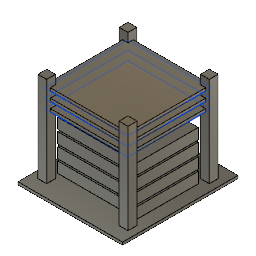
Mechanical Team Design 3Boards v2 (Autodesk Fusion 360 design; units mm, degrees)
Autodesk Fusion 360 part; units mm, degrees
box "BoxPrimitive1" add length 50 width 50 height 50 placed x (0, 0, 1) y (1, 0, 0) z (0, 1, 0) at (-20, 0, 10) makes body 1
box "BoxPrimitive2" add length 1.6 width 58 height 64 placed x (0, 0, -1) y (-1, 0, 0) z (0, 1, 0) at (33, 0, -10) separate body makes body 2
move_face "MoveFace1" by (10, 0, 0) 2 faces at (13.6667, 21.3333, -10) (-5.6667, 0, -10.5333) on bodies 2
move_body "Move1" bodies 2 to x (1, 0, 0) y (0, 1, 0) z (0, 0, 1) at (0, 0, 20)
move_face "MoveFace2" by (0, 5, 0) 1 faces at (13.6667, 21.3333, 10) on bodies 2
move_body "Move2" bodies 2 to x (1, 0, 0) y (0, 1, 0) z (0, 0, 1) at (0, -7, 0)
move_body "Move3" bodies 2 to x (1, 0, 0) y (0, 1, 0) z (0, 0, 1) at (5, 0, 0)
move_body "Move4" bodies 2 to x (1, 0, 0) y (0, 1, 0) z (0, 0, 1) at (-4, 0, 0)
sketch "Sketch4" plane through (0, 0, 10) normal (0, 0, 1) x (-1, 0, 0)
  line L0 (24, -57) -> (24, 7)
  line L1 (24, 7) -> (-34, 7)
  line L2 (-34, 7) -> (-34, -57)
  line L3 (-34, -57) -> (24, -57)
  line L4 (20, 0) -> (15, 0)
  line L5 (15, 0) -> (15, -5)
  line L6 (15, -5) -> (20, -5)
  line L7 (20, -5) -> (20, 0)
  line L8 (-5, -50) -> (-5, 0)
  line L9 (20, -25) -> (-30, -25)
  line L10 (15, -45) -> (20, -45)
  line L11 (20, -45) -> (20, -50)
  line L12 (15, -50) -> (15, -45)
  line L13 (20, -50) -> (15, -50)
  line L14 (-30, -50) -> (-25, -50)
  line L15 (-30, -45) -> (-30, -50)
  line L16 (-25, -50) -> (-25, -45)
  line L17 (-25, -45) -> (-30, -45)
  line L18 (-25, -5) -> (-30, -5)
  line L19 (-25, 0) -> (-25, -5)
  line L20 (-30, 0) -> (-25, 0)
  line L21 (-30, -5) -> (-30, 0)
  constraint horizontal L4
  constraint vertical L5
  constraint horizontal L6
  constraint vertical L7
  constraint perpendicular L4 L8
  constraint perpendicular L0 L9
  constraint symmetric L4.start L9 L11.end
  constraint symmetric L4.end L9 L12.start
  constraint symmetric L5.end L9 L10.start
  constraint symmetric L6.end L9 L10.end
  constraint symmetric L4.start L8 L20.start
  constraint symmetric L4.end L8 L19.start
  constraint symmetric L5.end L8 L18.start
  constraint symmetric L6.end L8 L18.end
  constraint symmetric L8 L10.start L16.end
  constraint symmetric L8 L10.end L15.start
  constraint symmetric L8 L11.end L14.start
  constraint symmetric L8 L12.start L14.end
extrude "Extrude1" add sketch "Sketch4" along normal blind 50 contours L4 L5 L6 L7 | L10 L11 L12 L13 | L14 L15 L16 L17 | L18 L19 L20 L21 bodies 2
ref_plane "WorkPlane1" through (0, 0, 53.4) normal (0, 0, 1) x (1, 0, 0)
sketch "Sketch6" plane through (0, 0, 53.4) normal (0, 0, 1) x (1, 0, 0)
  line L0 (28, 2) -> (-18, 2)
  line L1 (-18, 2) -> (-18, 48)
  line L2 (-18, 48) -> (28, 48)
  line L3 (28, 48) -> (28, 2)
  constraint horizontal L0
  constraint vertical L1
  constraint horizontal L2
  constraint vertical L3
extrude "Extrude2" cut sketch "Sketch6" along normal blind 1.6 bodies 2
extrude "Extrude3" add sketch "Sketch6" along normal blind 1.6 bodies 2
ref_plane "WorkPlane2" through (0, 0, 48.4) normal (0, 0, 1) x (1, 0, 0)
sketch "Sketch8" plane through (0, 0, 48.4) normal (0, 0, 1) x (1, 0, 0)
  line L0 (-18, 2) -> (28, 2)
  line L1 (28, 2) -> (28, 48)
  line L2 (28, 48) -> (-18, 48)
  line L3 (-18, 48) -> (-18, 2)
  constraint horizontal L0
  constraint vertical L1
  constraint horizontal L2
  constraint vertical L3
extrude "Extrude4" cut sketch "Sketch8" along normal blind 1.6 bodies 2
extrude "Extrude5" add sketch "Sketch8" along normal blind 1.6 bodies 2
ref_plane "WorkPlane3" through (0, 0, 43.4) normal (0, 0, 1) x (1, 0, 0)
sketch "Sketch9" plane through (0, 0, 43.4) normal (0, 0, 1) x (1, 0, 0)
  line L0 (-18, 2) -> (28, 2)
  line L1 (28, 2) -> (28, 48)
  line L2 (28, 48) -> (-18, 48)
  line L3 (-18, 48) -> (-18, 2)
  constraint horizontal L0
  constraint vertical L1
  constraint horizontal L2
  constraint vertical L3
extrude "Extrude6" cut sketch "Sketch9" along normal blind 1.6 bodies 2
extrude "Extrude7" add sketch "Sketch9" along normal blind 1.6 bodies 2
ref_plane "WorkPlane4" through (5, 25, 10) normal (0, 0, 1) x (0, 1, 0)
sketch "Sketch11" plane through (5, 25, 10) normal (0, 0, 1) x (1, 0, 0)
  line L0 (-22, 17) -> (22, 17)
  line L1 (22, 17) -> (22, -17)
  line L2 (22, -17) -> (-22, -17)
  line L3 (-22, -17) -> (-22, 17)
  constraint horizontal L0
  constraint vertical L1
  constraint horizontal L2
  constraint vertical L3
extrude "Extrude8" add sketch "Sketch11" along normal blind 6 bodies 2
ref_plane "WorkPlane5" through (5, 25, 17) normal (0, 0, 1) x (1, 0, 0)
sketch "Sketch12" plane through (5, 25, 17) normal (0, 0, 1) x (1, 0, 0)
  line L0 (-22, 17) -> (22, 17)
  line L1 (22, 17) -> (22, -17)
  line L2 (22, -17) -> (-22, -17)
  line L3 (-22, -17) -> (-22, 17)
  constraint horizontal L0
  constraint vertical L1
  constraint horizontal L2
  constraint vertical L3
extrude "Extrude9" add sketch "Sketch12" along normal blind 6 bodies 2 makes body 3
ref_plane "WorkPlane6" through (5, 25, 24) normal (0, 0, 1) x (1, 0, 0)
sketch "Sketch13" plane through (5, 25, 24) normal (0, 0, 1) x (1, 0, 0)
  line L0 (-22, 17) -> (22, 17)
  line L1 (22, 17) -> (22, -17)
  line L2 (22, -17) -> (-22, -17)
  line L3 (-22, -17) -> (-22, 17)
  constraint horizontal L0
  constraint vertical L1
  constraint horizontal L2
  constraint vertical L3
extrude "Extrude10" add sketch "Sketch13" along normal blind 6 separate body makes body 4
ref_plane "WorkPlane7" through (5, 25, 31) normal (0, 0, 1) x (1, 0, 0)
sketch "Sketch14" plane through (5, 25, 31) normal (0, 0, 1) x (1, 0, 0)
  line L0 (-22, 17) -> (22, 17)
  line L1 (22, 17) -> (22, -17)
  line L2 (22, -17) -> (-22, -17)
  line L3 (-22, -17) -> (-22, 17)
  constraint horizontal L0
  constraint vertical L1
  constraint horizontal L2
  constraint vertical L3
extrude "Extrude11" add sketch "Sketch14" along normal blind 6 separate body makes body 5
hidden bodies 1
equation "d31 = 10 mm + 50 mm - 5 mm - 1.6 mm"
equation "d36 = 10 mm + 50 mm - 10 mm - 1.6 mm"
equation "d41 = 10 mm + 50 mm - 1.6 mm - 15 mm"
